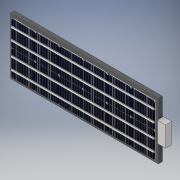
# Autodesk Inventor part: Solar_panel1
Saved by Autodesk Inventor 2018 (Build 220112000, 112)
## iProperties
Created: 2021-03-13
Part Number: Solar_panel1
Material: Generic
Document SubType Name: Modeling
Designer: Patel
Density: 1 g/cm^3
Appearance: Default
Author: Patel
Autodesk Inventor part; units mm, degrees
ref_plane "YZ Plane" through (0, 0, 0) normal (1, 0, 0) x (0, 1, 0)
ref_plane "XZ Plane" through (0, 0, 0) normal (0, 1, 0) x (-1, 0, 0)
ref_plane "XY Plane" through (0, 0, 0) normal (0, 0, 1) x (1, 0, 0)
sketch "Sketch1" plane through (0, 0, 0) normal (0, 0, 1) x (1, 0, 0)
  line L0 (-177.5, 65) -> (177.5, 65)
  line L1 (177.5, 65) -> (177.5, -65)
  line L2 (177.5, -65) -> (-177.5, -65)
  line L3 (-177.5, -65) -> (-177.5, 65)
  line L4 (-177.5, 65) -> (177.5, -65) construction
  line L5 (177.5, 65) -> (-177.5, -65) construction
  point P0 (0, 0)
  dimension "d0" = 355
  dimension "d1" = 130
  constraints: 12 end point, 2 midpoint, 2 parallel, 1 horizontal, 1 perpendicular
  measures "d0" distance of L1.end L2.end
  measures "d1" distance of L0.end L1.end
extrude "Extrusion1" add sketch "Sketch1" along normal mid plane 10
sketch "Sketch2" plane through (0, 0, 5) normal (0, 0, 1) x (1, 0, 0)
  line L0 (-172.5, 63) -> (-122.5, 63)
  line L1 (-118.5, 59) -> (-118.5, 4.5)
  line L2 (-122.5, 0.5) -> (-172.5, 0.5)
  line L3 (-176.5, 4.5) -> (-176.5, 59)
  line L4 (177.5, 65) -> (-177.5, 65) projected
  line L5 (-177.5, 65) -> (-177.5, -65) projected
  arc A0 (-172.5, 63) -> (-176.5, 59) centre (-172.5, 59) ccw
  arc A1 (-118.5, 59) -> (-122.5, 63) centre (-122.5, 59) ccw
  arc A2 (-122.5, 0.5) -> (-118.5, 4.5) centre (-122.5, 4.5) ccw
  arc A3 (-176.5, 4.5) -> (-172.5, 0.5) centre (-172.5, 4.5) ccw
  point P0 (0, 0)
  point P1 (-118.5, 0.5)
  point P2 (-118.5, 63)
  point P3 (-176.5, 0.5)
  dimension "d4" = 58
  dimension "d5" = 62.5
  dimension "d6" = 2
  dimension "d7" = 1
  dimension "d8" = 4
  constraints: 8 end point, 8 point on circle, 8 tangent, 6 point on line, 4 centre point, 3 equal radius, 2 parallel, 1 horizontal, 1 perpendicular
  measures "d4" distance of point (-118.5, 0.5) point (-176.5, 0.5)
  measures "d5" distance of point (-118.5, 63) point (-118.5, 0.5)
  measures "d6" distance between parallel lines of L4 L0
  measures "d7" distance between parallel lines of L5 L3
  measures "d8" radius of A0
extrude "Extrusion2" add sketch "Sketch2" along normal blind 3
pattern_linear "Rectangular Pattern1" count 6 spacing 59 along (1, 0, 0) of "Extrusion2"
pattern_linear "Rectangular Pattern2" count 2 spacing 63.5 along (0, -1, 0) of "Extrusion2", "Rectangular Pattern1"
sketch "Sketch3" plane through (0, 0, 8) normal (0, 0, 1) x (1, 0, 0)
  line L0 (-122.5, 63) -> (-172.5, 63) projected
  line L1 (-172, 63) -> (-172, -63)
  line L2 (-172.5, -63) -> (-122.5, -63) projected
  line L3 (-172, 63) -> (-46, 63) construction
  line L4 (-176.5, 59) -> (-176.5, 4.5) projected
  line L5 (-171, -63) -> (-171, 63)
  line L6 (-171, -63) -> (-45, -63) construction
  line L7 (-172, 63) -> (-171, 63)
  line L8 (-172, -63) -> (-171, -63)
  point P0 (0, 0)
  dimension "d17" = 126
  dimension "d18" = 90
  dimension "d19" = 4.5
  dimension "d20" = 126
  dimension "d21" = 90
  dimension "d22" = 1
  constraints: 12 end point, 6 perpendicular, 2 horizontal, 2 point on line
  measures "d17" distance of L1.start L1.end
  measures "d18" angle of L1 L3
  measures "d19" distance between parallel lines of L4 L1
  measures "d20" distance of L5.start L5.end
  measures "d21" angle of L6 L5
  measures "d22" distance between parallel lines of L5 L1
extrude "Extrusion3" cut sketch "Sketch3" against normal blind 1
pattern_linear "Rectangular Pattern3" count 13 spacing 4 along (1, 0, 0) of "Extrusion3"
pattern_linear "Rectangular Pattern4" count 6 spacing 59 along (1, 0, 0) of "Extrusion2", "Extrusion3", "Rectangular Pattern3"
sketch "Sketch4" plane through (0, 0, 8) normal (0, 0, 1) x (1, 0, 0)
  line L0 (-176.5, 59) -> (-176.5, 4.5) projected
  line L1 (-176.5, 48) -> (176.5, 48)
  line L2 (176.5, 48) -> (176.5, 44)
  line L3 (176.5, 44) -> (-176.5, 44)
  line L4 (-176.5, 44) -> (-176.5, 48)
  line L5 (-168, 63) -> (-171, 63) projected
  line L6 (-176.5, 19.5) -> (176.5, 19.5)
  line L7 (176.5, 15.5) -> (-176.5, 15.5)
  line L8 (176.5, 19.5) -> (176.5, 15.5)
  line L9 (-176.5, 15.5) -> (-176.5, 19.5)
  point P0 (0, 0)
  dimension "d31" = 353
  dimension "d32" = 4
  dimension "d33" = 15
  dimension "d36" = 28.5
  constraints: 16 end point, 2 parallel, 1 horizontal, 1 perpendicular, 1 point on line, 1 vertical, 8 other
  measures "d31" distance of L2.end L3.end
  measures "d32" distance of L1.end L2.end
  measures "d33" distance between parallel lines of L5 L1
  measures "d36" distance of L1.start L6.start
extrude "Extrusion4" add sketch "Sketch4" along normal blind 2 separate body
pattern_linear "Rectangular Pattern5" count 2 spacing 63 along (0, -1, 0) of "Extrusion4" bodies 2
sketch "Sketch5" plane through (0, 0, 5) normal (0, 0, 1) x (1, 0, 0)
  line L0 (-177.5, -65) -> (177.5, -65) projected
  line L1 (-177.5, 65) -> (177.5, 65)
  line L2 (177.5, 65) -> (177.5, -65)
  line L3 (177.5, -65) -> (-177.5, -65)
  line L4 (-177.5, -65) -> (-177.5, 65)
  line L5 (182.5, 70) -> (-182.5, 70)
  line L6 (-182.5, 70) -> (-182.5, -70)
  line L7 (-182.5, -70) -> (182.5, -70)
  line L8 (182.5, -70) -> (182.5, 70)
  point P0 (0, 0)
  dimension "d46" = 5
  constraints: 16 end point, 4 parallel, 2 perpendicular, 1 horizontal, 3 other
  measures "d46" distance between parallel lines of L1 L5
extrude "Extrusion5" add sketch "Sketch5" against normal blind 10 bodies 1
sketch "Sketch6" plane through (0, 0, 0) normal (0, 0, 1) x (1, 0, 0)
  line L0 (182.5, 25) -> (202.8692, 25)
  line L1 (202.8692, 25) -> (202.8692, -25)
  line L2 (202.8692, -25) -> (182.5, -25)
  line L3 (182.5, -25) -> (182.5, 25)
  point P0 (0, 0)
  dimension "d49" = 50
  dimension "d50" = 20.3692
  dimension "d51" = 202.8692
  dimension "d52" = 25
  constraints: 8 end point, 2 parallel, 1 horizontal, 1 perpendicular
  measures "d49" distance of L0.end L1.end
  measures "d50" distance between parallel lines of L1 L3
  measures "d51" distance from line of point (0, 0) L1
  measures "d52" distance from line of point (0, 0) L0
extrude "Extrusion6" add sketch "Sketch6" along normal mid plane 15 separate body
sketch "Sketch7" plane through (0, 0, 5) normal (0, 0, 1) x (1, 0, 0)
  point P0 (0, 0)
body "Solid1"
body "Solid2"
body "Solid3"
